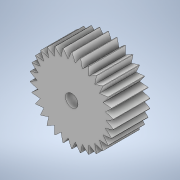
# Autodesk Inventor part: gear(1.5 inch with 2mm extra)
Saved by Autodesk Inventor 2022 (Build 260153000, 153)
## iProperties
Created: 2021-07-10
Part Number: gear(1.5 inch with 2mm extra)
Material: Generic
Document SubType Name: Modeling
Designer: hp
Density: 1 g/cm^3
Appearance: Default
Author: hp
Autodesk Inventor part; units mm, degrees
ref_plane "YZ Plane" through (0, 0, 0) normal (1, 0, 0) x (0, 1, 0)
ref_plane "XZ Plane" through (0, 0, 0) normal (0, 1, 0) x (-1, 0, 0)
ref_plane "XY Plane" through (0, 0, 0) normal (0, 0, 1) x (1, 0, 0)
sketch "Sketch1" plane through (0, 0, 0) normal (0, 0, 1) x (1, 0, 0)
  circle A0 centre (0, 0) radius 20.05
  dimension "d0" = 40.1
  constraints: 1 centre point, 1 coincident
  measures "d0" diameter of A0
extrude "Extrusion1" add sketch "Sketch1" along normal blind 17.5
sketch "Sketch2" plane through (0, 0, 17.5) normal (0, 0, 1) x (1, 0, 0)
  line L0 (-16.51, 0) -> (-20.1782, -2.1178)
  line L1 (-20.1782, -2.1178) -> (-20.1782, 2.1178)
  line L2 (-20.1782, 2.1178) -> (-16.51, 0)
  line L3 (-16.1492, -3.4326) -> (-19.297, -6.2669)
  line L4 (-19.297, -6.2669) -> (-20.1776, -2.1237)
  line L5 (-20.1776, -2.1237) -> (-16.1492, -3.4326)
  line L6 (-15.0827, -6.7152) -> (-17.5723, -10.142)
  line L7 (-17.5723, -10.142) -> (-19.2951, -6.2725)
  line L8 (-19.2951, -6.2725) -> (-15.0827, -6.7152)
  line L9 (-13.3569, -9.7043) -> (-15.0797, -13.5738)
  line L10 (-15.0797, -13.5738) -> (-17.5694, -10.1471)
  line L11 (-17.5694, -10.1471) -> (-13.3569, -9.7043)
  line L12 (-11.0474, -12.2693) -> (-11.928, -16.4125)
  line L13 (-11.928, -16.4125) -> (-15.0757, -13.5782)
  line L14 (-15.0757, -13.5782) -> (-11.0474, -12.2693)
  line L15 (-8.255, -14.2981) -> (-8.255, -18.5338)
  line L16 (-8.255, -18.5338) -> (-11.9232, -16.4159)
  line L17 (-11.9232, -16.4159) -> (-8.255, -14.2981)
  line L18 (-5.1019, -15.702) -> (-4.2212, -19.8451)
  line L19 (-4.2212, -19.8451) -> (-8.2496, -18.5362)
  line L20 (-8.2496, -18.5362) -> (-5.1019, -15.702)
  line L21 (-1.7258, -16.4196) -> (-0.003, -20.2891)
  line L22 (-0.003, -20.2891) -> (-4.2154, -19.8463)
  line L23 (-4.2154, -19.8463) -> (-1.7258, -16.4196)
  line L24 (1.7258, -16.4196) -> (4.2154, -19.8463)
  line L25 (4.2154, -19.8463) -> (0.003, -20.2891)
  line L26 (0.003, -20.2891) -> (1.7258, -16.4196)
  line L27 (5.1019, -15.702) -> (8.2496, -18.5362)
  line L28 (8.2496, -18.5362) -> (4.2212, -19.8451)
  line L29 (4.2212, -19.8451) -> (5.1019, -15.702)
  line L30 (8.255, -14.2981) -> (11.9232, -16.4159)
  line L31 (11.9232, -16.4159) -> (8.255, -18.5338)
  line L32 (8.255, -18.5338) -> (8.255, -14.2981)
  line L33 (11.0474, -12.2693) -> (15.0757, -13.5782)
  line L34 (15.0757, -13.5782) -> (11.928, -16.4125)
  line L35 (11.928, -16.4125) -> (11.0474, -12.2693)
  line L36 (13.3569, -9.7043) -> (17.5694, -10.1471)
  line L37 (17.5694, -10.1471) -> (15.0797, -13.5738)
  line L38 (15.0797, -13.5738) -> (13.3569, -9.7043)
  line L39 (15.0827, -6.7152) -> (19.2951, -6.2725)
  line L40 (19.2951, -6.2725) -> (17.5723, -10.142)
  line L41 (17.5723, -10.142) -> (15.0827, -6.7152)
  line L42 (16.1492, -3.4326) -> (20.1776, -2.1237)
  line L43 (20.1776, -2.1237) -> (19.297, -6.2669)
  line L44 (19.297, -6.2669) -> (16.1492, -3.4326)
  line L45 (16.51, 0) -> (20.1782, 2.1178)
  line L46 (20.1782, 2.1178) -> (20.1782, -2.1178)
  line L47 (20.1782, -2.1178) -> (16.51, 0)
  line L48 (16.1492, 3.4326) -> (19.297, 6.2669)
  line L49 (19.297, 6.2669) -> (20.1776, 2.1237)
  line L50 (20.1776, 2.1237) -> (16.1492, 3.4326)
  line L51 (15.0827, 6.7152) -> (17.5723, 10.142)
  line L52 (17.5723, 10.142) -> (19.2951, 6.2725)
  line L53 (19.2951, 6.2725) -> (15.0827, 6.7152)
  line L54 (13.3569, 9.7043) -> (15.0797, 13.5738)
  line L55 (15.0797, 13.5738) -> (17.5694, 10.1471)
  line L56 (17.5694, 10.1471) -> (13.3569, 9.7043)
  line L57 (11.0474, 12.2693) -> (11.928, 16.4125)
  line L58 (11.928, 16.4125) -> (15.0757, 13.5782)
  line L59 (15.0757, 13.5782) -> (11.0474, 12.2693)
  line L60 (8.255, 14.2981) -> (8.255, 18.5338)
  line L61 (8.255, 18.5338) -> (11.9232, 16.4159)
  line L62 (11.9232, 16.4159) -> (8.255, 14.2981)
  line L63 (5.1019, 15.702) -> (4.2212, 19.8451)
  line L64 (4.2212, 19.8451) -> (8.2496, 18.5362)
  line L65 (8.2496, 18.5362) -> (5.1019, 15.702)
  line L66 (1.7258, 16.4196) -> (0.003, 20.2891)
  line L67 (0.003, 20.2891) -> (4.2154, 19.8463)
  line L68 (4.2154, 19.8463) -> (1.7258, 16.4196)
  line L69 (-1.7258, 16.4196) -> (-4.2154, 19.8463)
  line L70 (-4.2154, 19.8463) -> (-0.003, 20.2891)
  line L71 (-0.003, 20.2891) -> (-1.7258, 16.4196)
  line L72 (-5.1019, 15.702) -> (-8.2496, 18.5362)
  line L73 (-8.2496, 18.5362) -> (-4.2212, 19.8451)
  line L74 (-4.2212, 19.8451) -> (-5.1019, 15.702)
  line L75 (-8.255, 14.2981) -> (-11.9232, 16.4159)
  line L76 (-11.9232, 16.4159) -> (-8.255, 18.5338)
  line L77 (-8.255, 18.5338) -> (-8.255, 14.2981)
  line L78 (-11.0474, 12.2693) -> (-15.0757, 13.5782)
  line L79 (-15.0757, 13.5782) -> (-11.928, 16.4125)
  line L80 (-11.928, 16.4125) -> (-11.0474, 12.2693)
  line L81 (-13.3569, 9.7043) -> (-17.5694, 10.1471)
  line L82 (-17.5694, 10.1471) -> (-15.0797, 13.5738)
  line L83 (-15.0797, 13.5738) -> (-13.3569, 9.7043)
  line L84 (-15.0827, 6.7152) -> (-19.2951, 6.2725)
  line L85 (-19.2951, 6.2725) -> (-17.5723, 10.142)
  line L86 (-17.5723, 10.142) -> (-15.0827, 6.7152)
  line L87 (-16.1492, 3.4326) -> (-20.1776, 2.1237)
  line L88 (-20.1776, 2.1237) -> (-19.297, 6.2669)
  line L89 (-19.297, 6.2669) -> (-16.1492, 3.4326)
  point P0 (0, 0)
  point P1 (-18.9555, 0)
  point P2 (-18.5413, -3.9411)
  point P3 (-17.3167, -7.7099)
  point P4 (-15.3353, -11.1418)
  point P5 (-12.6837, -14.0867)
  point P6 (-9.4777, -16.4159)
  point P7 (-5.8576, -18.0277)
  point P8 (-1.9814, -18.8517)
  point P9 (1.9814, -18.8517)
  point P10 (5.8576, -18.0277)
  point P11 (9.4777, -16.4159)
  point P12 (12.6837, -14.0867)
  point P13 (15.3353, -11.1418)
  point P14 (17.3167, -7.7099)
  point P15 (18.5413, -3.9411)
  point P16 (18.9555, 0)
  point P17 (18.5413, 3.9411)
  point P18 (17.3167, 7.7099)
  point P19 (15.3353, 11.1418)
  point P20 (12.6837, 14.0867)
  point P21 (9.4777, 16.4159)
  point P22 (5.8576, 18.0277)
  point P23 (1.9814, 18.8517)
  point P24 (-1.9814, 18.8517)
  point P25 (-5.8576, 18.0277)
  point P26 (-9.4777, 16.4159)
  point P27 (-12.6837, 14.0867)
  point P28 (-15.3353, 11.1418)
  point P29 (-17.3167, 7.7099)
  point P30 (-18.5413, 3.9411)
  dimension "d5" = 360
  constraints: 180 end point, 218 other
extrude "Extrusion2" cut sketch "Sketch2" against normal through all
sketch "Sketch3" plane through (0, 0, 0) normal (0, 0, -1) x (-1, 0, 0)
  point P0 (0, 0)
  point P1 (0, 0)
  constraints: 1 coincident
hole "Hole1" at (0, 0, 0) at (0, 0, 0) direction (0, 0, 1) diameter 6 end through all
body "Solid1"
